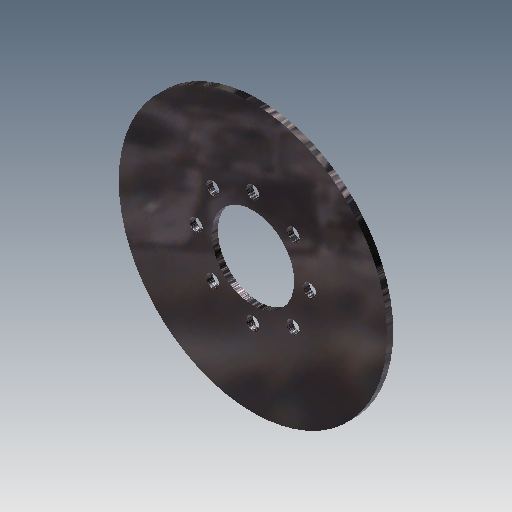
# Autodesk Inventor part: 先端アームパーツA
Saved by Autodesk Inventor 2019.4 (Build 234330000, 330)
## iProperties
Created: 2018-08-09
Part Number: 先端アームパーツA
Material: アルミニウム 6061
Document SubType Name: Modeling
Designer: Owner
Density: 2.7 g/cm^3
Appearance: アルミニウム - フラット
Mass: 30.949 g
Surface Area: 89.49 cm^2
Volume: 11.4626 cm^3
Author: Owner
Autodesk Inventor part; units mm, degrees
ref_plane "YZ Plane" through (0, 0, 0) normal (1, 0, 0) x (0, 1, 0)
ref_plane "XZ Plane" through (0, 0, 0) normal (0, 1, 0) x (-1, 0, 0)
ref_plane "XY Plane" through (0, 0, 0) normal (0, 0, 1) x (1, 0, 0)
sketch "スケッチ1" plane through (0, 0, 0) normal (0, 0, 1) x (1, 0, 0)
  line L0 (25, -23) -> (-25, -23) construction
  line L1 (25, 23) -> (25, -23) construction
  line L2 (-25, 23) -> (25, 23) construction
  arc A0 (8.5, 1.9365) -> (7.0484, 3.4357) centre (7, 1.9365) ccw construction
  line L3 (8.5, 1.9365) -> (8.5, -1.9365) construction
  arc A1 (7.0484, -3.4357) -> (8.5, -1.9365) centre (7, -1.9365) ccw construction
  arc A2 (2.9516, -3.4357) -> (7.0484, -3.4357) centre (5, 0) ccw construction
  arc A3 (1.5, -1.9365) -> (2.9516, -3.4357) centre (3, -1.9365) ccw construction
  line L4 (1.5, -1.9365) -> (1.5, 1.9365) construction
  arc A4 (2.9516, 3.4357) -> (1.5, 1.9365) centre (3, 1.9365) ccw construction
  arc A5 (7.0484, 3.4357) -> (2.9516, 3.4357) centre (5, 0) ccw construction
  circle A6 centre (5, 0) radius 27.5 construction
  circle A7 centre (5, 0) radius 15.5 construction
  circle A8 centre (5, 0) radius 13.75 construction
  line L5 (25, 14) -> (25, 23) construction
  line L6 (-275, 23) -> (25, 23) construction
  line L7 (-275, 23) -> (-275, 14) projected
  line L8 (-275, 14) -> (25, 14) construction
  line L9 (25, -23) -> (25, -14) construction
  line L10 (-275, -14) -> (25, -14) construction
  line L11 (-275, -14) -> (-275, -23) projected
  line L12 (-275, -23) -> (25, -23) construction
  circle A9 centre (18.75, 0) radius 1.6
  circle A10 centre (14.7227, 9.7227) radius 1.6
  circle A11 centre (5, 13.75) radius 1.6
  circle A12 centre (-4.7227, 9.7227) radius 1.6
  circle A13 centre (-8.75, 0) radius 1.6
  circle A14 centre (-4.7227, -9.7227) radius 1.6
  circle A15 centre (5, -13.75) radius 1.6
  circle A16 centre (14.7227, -9.7227) radius 1.6
  circle A17 centre (5, 0) radius 10
  circle A18 centre (5, 0) radius 32.5
  point P0 (0, 0)
  dimension "d3" = 27.5
  dimension "d1" = 55
  dimension "d2" = 31
  dimension "d4" = 3.2
  dimension "d7" = 360
  dimension "d9" = 20
  dimension "d12" = 65
  constraints: 12 centre point, 3 coincident, 1 horizontal alignment, 19 other
  measures "d1" diameter of A6
  measures "d2" diameter of A7
  measures "d4" diameter of A9
  measures "d9" diameter of A17
  measures "d12" diameter of A18
extrude "押し出し1" add sketch "スケッチ1" along normal blind 1.5
